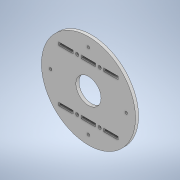
# Autodesk Inventor part: Base4
Saved by Autodesk Inventor 2022 (Build 260153000, 153)
## iProperties
Created: 2021-09-09
Part Number: Base4
Material: Generic
Document SubType Name: Modeling
Designer: Administrador
Density: 1 g/cm^3
Appearance: Default
Author: Administrador
Autodesk Inventor part; units mm, degrees
ref_plane "YZ Plane" through (0, 0, 0) normal (1, 0, 0) x (0, 1, 0)
ref_plane "XZ Plane" through (0, 0, 0) normal (0, 1, 0) x (-1, 0, 0)
ref_plane "XY Plane" through (0, 0, 0) normal (0, 0, 1) x (1, 0, 0)
sketch "Sketch3" plane through (0, 0, 0) normal (0, 0, 1) x (1, 0, 0)
  circle A0 centre (0, 0) radius 46
  circle A1 centre (0, 0) radius 12.3
  circle A2 centre (0, 0) radius 37 construction
  circle A3 centre (0, 37) radius 1.25
  circle A4 centre (37, 0) radius 1.25
  circle A5 centre (0, -37) radius 1.25
  circle A6 centre (-37, 0) radius 1.25
  line L0 (-11, 25.5) -> (-11, -25.5) construction
  circle A7 centre (-11, 25.5) radius 1.55
  circle A8 centre (-11, -25.5) radius 1.55
  circle A9 centre (11, -25.5) radius 1.55
  line L1 (7, -27.05) -> (-7, -27.05)
  line L2 (-7, -27.05) -> (-7, -24.05)
  line L3 (-7, -24.05) -> (7, -24.05)
  line L4 (7, -24.05) -> (7, -27.05)
  line L5 (-15, -27.05) -> (-29, -27.05)
  line L6 (-29, -27.05) -> (-29, -24.05)
  line L7 (-29, -24.05) -> (-15, -24.05)
  line L8 (-15, -24.05) -> (-15, -27.05)
  line L9 (15, -27.05) -> (29, -27.05)
  line L10 (29, -27.05) -> (29, -24.05)
  line L11 (29, -24.05) -> (15, -24.05)
  line L12 (15, -24.05) -> (15, -27.05)
  line L13 (18.1239, 27.05) -> (15, 27.05)
  line L14 (7, 24) -> (-7, 24)
  line L15 (-7, 24) -> (-7, 27)
  line L16 (-7, 27) -> (7, 27)
  line L17 (7, 27) -> (7, 24)
  line L18 (-15, 24) -> (-29, 24)
  line L19 (-29, 24) -> (-29, 27)
  line L20 (-29, 27) -> (-15, 27)
  line L21 (-15, 27) -> (-15, 24)
  line L22 (15, 24) -> (29, 24)
  line L23 (29, 24) -> (29, 27)
  line L24 (29, 27) -> (15, 27)
  line L25 (15, 27) -> (15, 24)
  circle A10 centre (11, 25.5) radius 1.55
  line L26 (-46, -25.55) -> (46, -25.55) construction
  point P0 (46, 0)
  dimension "d74" = 92
  dimension "d32" = 2.5
  dimension "d33" = 2.5
  dimension "d34" = 2.5
  dimension "d35" = 2.5
  dimension "d45" = 3.1
  dimension "d46" = 3.1
  dimension "d47" = 3.1
  dimension "d50" = 14
  dimension "d51" = 4
  dimension "d53" = 14
  dimension "d54" = 4
  dimension "d57" = 14
  dimension "d58" = 14
  dimension "d59" = 14
  dimension "d60" = 3
  dimension "d61" = 14
  dimension "d64" = 3
  dimension "d65" = 3
  dimension "d71" = 1.5
  dimension "d72" = 1.5
  dimension "d75" = 74
  dimension "d78" = 24.6
  dimension "d80" = 3.1
  dimension "d81" = 25.5
  dimension "d82" = 25.5
  dimension "d83" = 22
  dimension "d84" = 11
  dimension "d87" = 4
  dimension "d91" = 22
  dimension "d92" = 1.5
  dimension "d93" = 1.5
  dimension "d94" = 1.5
  dimension "d95" = 1.5
  dimension "d96" = 1.5
  dimension "d97" = 1.5
  dimension "d98" = 4
  constraints: 54 end point, 12 parallel, 10 centre point, 8 horizontal, 6 perpendicular, 5 coincident, 4 point on circle, 1 horizontal alignment, 3 other
  measures "d32" diameter of A3
  measures "d33" diameter of A4
  measures "d34" diameter of A5
  measures "d35" diameter of A6
  measures "d45" diameter of A9
  measures "d46" diameter of A8
  measures "d47" diameter of A7
  measures "d50" distance of L2.end L3.end
  measures "d51" distance from line of L2 A8.centre
  measures "d53" distance of L6.end L7.end
  measures "d54" distance from line of L8 L0.end
  measures "d57" distance of L11.end L10.end
  measures "d58" distance of L16.start L17.start
  measures "d59" distance of L20.start L21.start
  measures "d60" distance between parallel lines of L20 L18
  measures "d61" distance of L24.end L24.start
  measures "d64" distance between parallel lines of L16 L14
  measures "d65" distance between parallel lines of L24 L22
  measures "d71" distance from line of L20 L0.start
  measures "d72" distance from line of L16 L0.start
  measures "d75" diameter of A2
  measures "d78" diameter of A1
  measures "d80" diameter of A10
  measures "d81" vertical distance of L0.start point (0, 0)
  measures "d82" vertical distance of A10.centre point (0, 0)
  measures "d83" distance of A10.centre L0.start
  measures "d84" horizontal distance of A7.centre A1.centre
  measures "d87" distance from line of L12 A9.centre
  measures "d91" distance of A9.centre A8.centre
  measures "d92" distance between parallel lines of L5 L26
  measures "d93" distance between parallel lines of L7 L26
  measures "d94" distance between parallel lines of L3 L26
  measures "d95" distance between parallel lines of L1 L26
  measures "d96" distance between parallel lines of L11 L26
  measures "d97" distance between parallel lines of L26 L9
  measures "d98" distance from line of A9.centre L4
extrude "Extrusion2" add sketch "Sketch3" along normal blind 3
body "Solid2"
